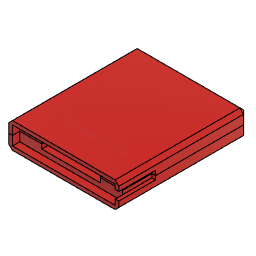
Mod (Autodesk Fusion 360 design; units mm, degrees)
Autodesk Fusion 360 part; units mm, degrees
note: some values were not read from the file. Chosen so that the rebuilt part matches the saved one: which face or edge a step refers to.
sketch "Skizze1" plane through (0, 0, 0) normal (0, 0, 1) x (1, 0, 0)
  line L0 (0, 0) -> (30, 0)
  line L1 (30, 0) -> (30, 35)
  line L2 (30, 35) -> (0, 35)
  line L3 (0, 35) -> (0, 0)
  line L4 (1.5, 1.5) -> (28.5, 1.5)
  line L5 (28.5, 1.5) -> (28.5, 33.5)
  line L6 (28.5, 33.5) -> (1.5, 33.5)
  line L7 (1.5, 33.5) -> (1.5, 1.5)
  line L8 (1.5, 1.5) -> (1.5, 0)
  line L9 (28.5, 1.5) -> (28.5, 0)
  dimension "d1" = 30
  dimension "d2" = 35
  dimension "d3" = -1.5
  constraint horizontal L0
  constraint vertical L1
  constraint horizontal L2
  constraint vertical L3
  constraint coincident L0.start L3.end
  constraint coincident L0 L8.end
  constraint perpendicular L0 L8
  constraint coincident L0 L9.end
  constraint perpendicular L0 L9
  measures "d1" distance of L0.start L0.end
  measures "d2" distance of L0.start L2.end
extrude "Extrusion1" add sketch "Skizze1" along normal blind 1 makes body 1
copy_body "Körper->Berechn1" bodies 1 removing the originals makes body 2 in component "Bottom"
extrude "Extrusion1'" add sketch "Skizze1" along normal blind 2.5 from surface at 1 contours L0 L1 L2 L3 L5 L6 L7 L8 L9 bodies 2 in component "Bottom"
sketch "Skizze1 (2)" plane through (0, 0, 1) normal (0, 0, 1) x (-1, 0, 0) in component "Bottom"
  line L0 (-1.5, -33.5) -> (-1.5, 0)
  line L1 (-1.5, 0) -> (-28.5, 0)
  line L2 (-28.5, 0) -> (-28.5, -33.5)
  line L3 (-28.5, -33.5) -> (-1.5, -33.5)
  line L4 (-1.5, 0) -> (-30.5, 0)
  line L5 (-30.5, 0) -> (-30.5, -9)
  line L6 (-30.5, -9) -> (-1.5, -9)
  line L7 (-1.5, -9) -> (-1.5, 0)
  dimension "d9" = 9
  constraint horizontal L4
  constraint vertical L5
  constraint horizontal L6
  constraint vertical L7
  constraint coincident L0.end L1.start
  measures "d9" distance of L0.end L6.end
extrude "Extrusion2" add sketch "Skizze1 (2)" along normal blind 1.3 contours L0 L1 L2 L4 L6 L7 bodies 2 in component "Bottom"
sketch "Skizze2" plane through (0, 0, 2.3) normal (0, 0, 1) x (-1, 0, 0) in component "Bottom"
  line L0 (-1.5, -9) -> (-1.5, 0)
  line L1 (-1.5, 0) -> (-28.5, 0)
  line L2 (-28.5, 0) -> (-28.5, -9)
  line L3 (-28.5, -9) -> (-1.5, -9)
  line L4 (-15, 0) -> (-15, -9) construction
  line L5 (-7, 0.6429) -> (-23, 0.6429)
  line L6 (-23, 0.6429) -> (-23, -9.6429)
  line L7 (-23, -9.6429) -> (-7, -9.6429)
  line L8 (-7, -9.6429) -> (-7, 0.6429)
  line L9 (-7, 0.6429) -> (-23, -9.6429) construction
  line L10 (-23, 0.6429) -> (-7, -9.6429) construction
  point P0 (-15, -4.5)
  dimension "d12" = 16
  constraint midpoint L1 L4.start
  constraint midpoint L3 L4.end
  constraint horizontal L5
  constraint perpendicular L5 L6
  constraint parallel L5 L7
  constraint parallel L6 L8
  constraint coincident L9 P0
  constraint coincident L10 P0
  constraint midpoint L4 P0
  measures "d12" distance of L6.end L7.end
extrude "Extrusion3" add sketch "Skizze2" along normal blind 1.2 contours L0 L1 L3 L8 | L1 L2 L3 L6 bodies 2 in component "Bottom"
sketch "Skizze2 (2)" plane through (0, 0, 0) normal (0, -1, 0) x (1, 0, 0)
  line L0 (0, 0) -> (30, 0)
  line L1 (30, 0) -> (30, 3.5)
  line L2 (30, 3.5) -> (23, 3.5)
  line L3 (23, 3.5) -> (23, 2.3)
  line L4 (23, 2.3) -> (7, 2.3)
  line L5 (7, 2.3) -> (7, 3.5)
  line L6 (7, 3.5) -> (0, 3.5)
  line L7 (0, 3.5) -> (0, 0)
  line L8 (1, 5.9237) -> (29, 5.9237)
  line L9 (29, 5.9237) -> (29, 1)
  line L10 (29, 1) -> (1, 1)
  line L11 (1, 1) -> (1, 5.9237)
  dimension "d15" = 1
  dimension "d16" = 1
  dimension "d17" = 1
  constraint horizontal L8
  constraint vertical L9
  constraint horizontal L10
  constraint vertical L11
  measures "d15" distance of L7 L11
  measures "d16" distance of L1 L9
  measures "d17" distance of L0 L10
extrude "Extrusion4" cut sketch "Skizze2 (2)" against normal blind 2 contours L2 L3 L4 L5 L6 L9 L10 L11 bodies 2 in component "Bottom"
chamfer "Fase1" distance 1 angle 45 5 edges at (0, 35, 1.75) (30, 35, 1.75) (30, 17.5, 0) (15, 35, 0) (0, 17.5, 0) on bodies 2 in component "Bottom"
mirror "Komponente spiegeln1" about plane through (0, 0, 0) normal (0, 0, 1) of bodies 2 makes body 3 in component "Top"
sketch "Skizze3" plane through (0, 0, 0) normal (0, -1, 0) x (1, 0, 0) in component "Bottom"
  line L0 (0, 1) -> (1, 0)
  line L1 (1, 0) -> (29, 0)
  line L2 (29, 0) -> (30, 1)
  line L3 (30, 1) -> (30, 3.5)
  line L4 (30, 3.5) -> (29, 3.5)
  line L5 (29, 3.5) -> (29, 1)
  line L6 (29, 1) -> (1, 1)
  line L7 (1, 1) -> (1, 3.5)
  line L8 (1, 3.5) -> (0, 3.5)
  line L9 (0, 3.5) -> (0, 1)
  line L10 (29, 3.5) -> (30, 3.5)
  line L11 (30, 3.5) -> (30, 2.5)
  line L12 (30, 2.5) -> (29, 2.5)
  line L13 (29, 2.5) -> (29, 3.5)
  dimension "d58" = 1
  constraint horizontal L10
  constraint vertical L11
  constraint horizontal L12
  constraint vertical L13
  constraint coincident L4.end L5.start
  measures "d58" distance of L4.end L12.end
extrude "Extrusion10" cut sketch "Skizze3" against normal blind 10 contours L3 L4 L5 L10 L11 L12 L13 bodies 2 in component "Bottom"
sketch "Skizze1 (3)" plane through (0, 0, 0) normal (0, -1, 0) x (1, 0, 0) in component "Top"
  line L0 (1, 0) -> (0, -1)
  line L1 (0, -1) -> (0, -3.5)
  line L2 (0, -3.5) -> (1, -3.5)
  line L3 (1, -3.5) -> (1, -1)
  line L4 (1, -1) -> (29, -1)
  line L5 (29, -1) -> (29, -3.5)
  line L6 (29, -3.5) -> (30, -3.5)
  line L7 (30, -3.5) -> (30, -1)
  line L8 (30, -1) -> (29, 0)
  line L9 (29, 0) -> (1, 0)
  line L10 (29, -3.5) -> (30, -3.5)
  line L11 (30, -3.5) -> (30, -2.25)
  line L12 (30, -2.25) -> (29, -2.25)
  line L13 (29, -2.25) -> (29, -3.5)
  constraint horizontal L10
  constraint vertical L11
  constraint horizontal L12
  constraint vertical L13
  constraint midpoint L7 L11.end
  constraint coincident L5.end L6.start
extrude "Extrusion1''" cut sketch "Skizze1 (3)" against normal blind 10 contours L5 L6 L7 L10 L11 L12 L13 bodies 3 in component "Top"
sketch "Skizze2 (3)" plane through (0, 0, -3.5) normal (0, 0, -1) x (1, 0, 0) in component "Top"
  line L0 (30, -10) -> (29, -10)
  line L1 (28.5, -9) -> (28.5, -33.5)
  line L2 (28.5, -33.5) -> (1.5, -33.5)
  line L3 (1.5, -33.5) -> (1.5, -9)
  line L4 (1, -2) -> (1, 0)
  line L5 (1, 0) -> (0, 0)
  line L6 (0, 0) -> (0, -34)
  line L7 (0, -34) -> (1, -35)
  line L8 (1, -35) -> (29, -35)
  line L9 (29, -35) -> (30, -34)
  line L10 (30, -34) -> (30, -10)
  line L11 (1.5, -9) -> (2.5, -9)
  line L12 (2.5, -9) -> (2.5, -38.5)
  line L13 (2.5, -38.5) -> (1.5, -38.5)
  line L14 (1.5, -38.5) -> (1.5, -9)
  line L15 (28.5, -9) -> (27.5, -9)
  line L16 (27.5, -9) -> (27.5, -38.5)
  line L17 (27.5, -38.5) -> (28.5, -38.5)
  line L18 (28.5, -38.5) -> (28.5, -9)
  line L19 (1.5, -33.5) -> (28.5, -33.5)
  line L20 (28.5, -33.5) -> (28.5, -32.5)
  line L21 (28.5, -32.5) -> (1.5, -32.5)
  line L22 (1.5, -32.5) -> (1.5, -33.5)
  line L23 (23, -2) -> (23, -9)
  line L24 (23, -9) -> (28.5, -9)
  line L25 (1.5, -9) -> (7, -9)
  line L26 (7, -9) -> (7, -2)
  line L27 (29, -10) -> (29, -2)
  line L28 (29, -2) -> (23, -2)
  line L29 (7, -2) -> (1, -2)
  dimension "d77" = 1
  dimension "d78" = 1
  dimension "d79" = 1
  constraint horizontal L11
  constraint vertical L12
  constraint horizontal L13
  constraint vertical L14
  constraint coincident L3.end L11.start
  constraint horizontal L15
  constraint vertical L16
  constraint horizontal L17
  constraint vertical L18
  constraint coincident L1.start L15.start
  constraint horizontal L19
  constraint vertical L20
  constraint horizontal L21
  constraint vertical L22
  constraint coincident L1 L20.end
  constraint coincident L2.end L3.start
  measures "d77" distance of L3.end L11.end
  measures "d78" distance of L1.start L15.end
  measures "d79" distance of L2.end L21.end
extrude "Extrusion3'" add sketch "Skizze2 (3)" along normal blind 1 and the other way blind 2.5 contours L1 L2 L16 L18 L19 L20 L21 | L1 L15 L16 L18 L21 L24 | L2 L12 L16 L19 L21 | L2 L3 L12 L14 L19 L21 L22 | L3 L11 L12 L14 L21 L25 bodies 3 in component "Top"
move_face "Flächen versetzen1" offset -0.5 5 faces at (28.1667, 9, -3.8333) (28.5, 17.1667, -3.8333) (2.1667, 9, -4.1667) (1.5, 25.3333, -3.8333) (10.5, 33.5, -4.1667) on bodies 3 in component "Top"
move_face "Flächen versetzen2" offset 0.5 3 faces at (27.5, 24.8333, -3) (19.1667, 32.5, -2.1667) (2.5, 24.8333, -3) on bodies 3 in component "Top"
sketch "Skizze3 (2)" plane through (0, 9, 0) normal (0, 1, 0) x (-1, 0, 0) in component "Top"
  line L0 (-27, -1) -> (-27, -3.5)
  line L1 (-27, -3.5) -> (-23, -3.5)
  line L2 (-23, -3.5) -> (-23, -2.3)
  line L3 (-23, -2.3) -> (-7, -2.3)
  line L4 (-7, -2.3) -> (-7, -3.5)
  line L5 (-7, -3.5) -> (-3, -3.5)
  line L6 (-3, -3.5) -> (-3, -1)
  line L7 (-3, -1) -> (-27, -1)
  line L8 (-3, -3.5) -> (-7, -3.5)
  line L9 (-7, -3.5) -> (-7, -1)
  line L10 (-7, -1) -> (-3, -1)
  line L11 (-3, -1) -> (-3, -3.5)
  line L12 (-23, -3.5) -> (-27, -3.5)
  line L13 (-27, -3.5) -> (-27, -1)
  line L14 (-27, -1) -> (-23, -1)
  line L15 (-23, -1) -> (-23, -3.5)
  constraint horizontal L8
  constraint vertical L9
  constraint horizontal L10
  constraint vertical L11
  constraint coincident L7 L9.end
  constraint coincident L5.end L6.start
  constraint horizontal L12
  constraint vertical L13
  constraint horizontal L14
  constraint vertical L15
  constraint coincident L0.start L7.end
  constraint coincident L1.end L2.start
extrude "Extrusion4'" add sketch "Skizze3 (2)" along normal blind 2 contours L0 L1 L2 L7 L12 L13 L14 L15 | L4 L5 L6 L7 L8 L9 L10 L11 bodies 3 in component "Top"
sketch "Skizze4" plane through (0, 9, 0) normal (0, 1, 0) x (-1, 0, 0) in component "Bottom"
  line L0 (-28.5, 1) -> (-1.5, 1)
  line L1 (-1.5, 1) -> (-1.5, 3.5)
  line L2 (-1.5, 3.5) -> (-7, 3.5)
  line L3 (-7, 3.5) -> (-7, 2.3)
  line L4 (-7, 2.3) -> (-23, 2.3)
  line L5 (-23, 2.3) -> (-23, 3.5)
  line L6 (-23, 3.5) -> (-28.5, 3.5)
  line L7 (-28.5, 3.5) -> (-28.5, 1)
  line L8 (-28.5, 3.5) -> (-23, 3.5)
  line L9 (-23, 3.5) -> (-23, 1)
  line L10 (-23, 1) -> (-28.5, 1)
  line L11 (-28.5, 1) -> (-28.5, 3.5)
  line L12 (-7, 3.5) -> (-1.5, 3.5)
  line L13 (-1.5, 3.5) -> (-1.5, 1)
  line L14 (-1.5, 1) -> (-7, 1)
  line L15 (-7, 1) -> (-7, 3.5)
  constraint horizontal L8
  constraint vertical L9
  constraint horizontal L10
  constraint vertical L11
  constraint coincident L0 L9.end
  constraint coincident L6.end L7.start
  constraint horizontal L12
  constraint vertical L13
  constraint horizontal L14
  constraint vertical L15
  constraint coincident L0.end L1.start
  constraint coincident L2.end L3.start
extrude "Extrusion13" add sketch "Skizze4" along normal blind 2 contours L0 L5 L6 L7 L8 L9 L10 L11 | L0 L1 L2 L3 L12 L13 L14 L15 bodies 2 in component "Bottom"
sketch "Skizze6" plane through (0, 9, 0) normal (0, 1, 0) x (-1, 0, 0)
  line L0 (-23, 6) -> (-23, 4.7)
  line L1 (-23, 4.7) -> (-7, 4.7)
  line L2 (-7, 4.7) -> (-7, 6)
  line L3 (-7, 6) -> (-23, 6)
extrude "Extrusion5" cut 2 faces at (27.6667, 9.5, -3.8333) (2.3333, 9.5, -3.8333) along direction (0, 1, 0) blind 1.5 on bodies 3 bodies 3 in component "Top"
component "Bottom" placed x (1, 0, 0) y (0, 1, 0) z (0, 0, 1) at (0, 0, 0)
component "Top" placed x (1, 0, 0) y (0, 1, 0) z (0, 0, 1) at (0, 0, 7)
